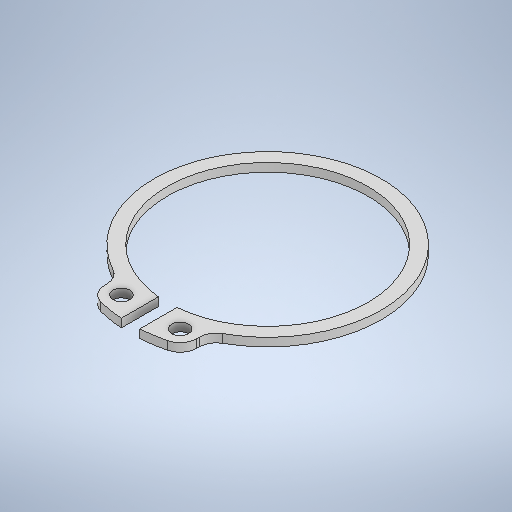
# Autodesk Inventor part: 49-01-002
Saved by Autodesk Inventor 2025.2 (Build 292293000, 293)
## iProperties
Created: 2024-11-28
Part Number: 49-01-002
Material: Generic
Document SubType Name: Modeling
Designer: Zvonko.Gabric
Density: 1 g/cm^3
Appearance: Default
Author: Zvonko.Gabric
Autodesk Inventor part; units mm, degrees
ref_plane "YZ Plane" through (0, 0, 0) normal (1, 0, 0) x (0, 1, 0)
ref_plane "XZ Plane" through (0, 0, 0) normal (0, 1, 0) x (-1, 0, 0)
ref_plane "XY Plane" through (0, 0, 0) normal (0, 0, 1) x (1, 0, 0)
sketch "Sketch1" plane through (0, 0, 0) normal (0, 1, 0) x (-1, 0, 0)
  line L0 (8.0103, 27.4413) -> (8.0103, 27.134)
  line L1 (12.4103, 25.424) -> (12.4103, 29.8377)
  circle A0 centre (10.0103, 27.4413) radius 1
  arc A1 (12.4103, 25.424) -> (13.5103, 1.5747) centre (13.5103, 13.5247) ccw
  arc A2 (6.9756, 25.3824) -> (13.5103, -0.0144) centre (13.5103, 13.5247) ccw
  arc A3 (6.9756, 25.3824) -> (8.0103, 27.134) centre (6.0103, 27.134) ccw
  arc A4 (9.5225, 29.3809) -> (8.0103, 27.4413) centre (10.0103, 27.4413) ccw
  arc A5 (12.4103, 29.8377) -> (9.5225, 29.3809) centre (13.5103, 13.5247) ccw
  line L2 (13.5103, 34.3082) -> (13.5103, -8.904)
  line L3 (19.0103, 27.4413) -> (19.0103, 27.134)
  line L4 (14.6103, 25.424) -> (14.6103, 29.8377)
  circle A6 centre (17.0103, 27.4413) radius 1
  arc A7 (13.5103, 1.5747) -> (14.6103, 25.424) centre (13.5103, 13.5247) ccw
  arc A8 (13.5103, -0.0144) -> (20.045, 25.3824) centre (13.5103, 13.5247) ccw
  arc A9 (19.0103, 27.134) -> (20.045, 25.3824) centre (21.0103, 27.134) ccw
  arc A10 (19.0103, 27.4413) -> (17.4981, 29.3809) centre (17.0103, 27.4413) ccw
  arc A11 (17.4981, 29.3809) -> (14.6103, 29.8377) centre (13.5103, 13.5247) ccw
  point P0 (0, 0)
  point P1 (12.4103, 27.6308)
  point P2 (14.6103, 27.6308)
  dimension "d0" = 11.95
  dimension "d1" = 13.5391
  dimension "d4" = 2.4
  dimension "d6" = 2
  dimension "d7" = 2
  dimension "d8" = 2
  constraints: 20 point on circle, 12 centre point, 10 end point, 8 symmetric about line, 2 point on line, 1 midpoint, 1 vertical, 6 other
  measures "d0" radius of A1
  measures "d1" radius of A2
  measures "d4" horizontal distance of point (12.41, 27.631) A0.centre
  measures "d6" radius of A3
  measures "d7" diameter of A0
  measures "d8" radius of A4
extrude "Extrusion1" add sketch "Sketch1" along normal blind 1
body "Solid1"
